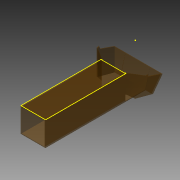
# Autodesk Inventor part: Ball Collector
Saved by Autodesk Inventor 2013 (Build 170138000, 138)
## iProperties
Created: 2014-09-14
Part Number: Ball Collector
Document SubType Name: Modeling
Designer: Family Room
Density: 1 g/cm^3
Material: Generic
Author: Family Room
Autodesk Inventor part; units mm, degrees
sketch "Sketch1" plane through (0, 0, 0) normal (0, 0, 1) x (1, 0, 0)
  line L0 (0, 0) -> (95.25, 0)
  line L1 (95.25, 0) -> (95.25, 95.25)
  line L2 (95.25, 95.25) -> (0, 95.25)
  line L3 (0, 95.25) -> (0, 0)
  line L4 (-3.175, -3.175) -> (98.425, -3.175)
  line L5 (98.425, -3.175) -> (98.425, 98.425)
  line L6 (98.425, 98.425) -> (-3.175, 98.425)
  line L7 (-3.175, 98.425) -> (-3.175, -3.175)
  dimension "d0" = 95.25
  dimension "d1" = 95.25
  dimension "d2" = 3.175
  constraints: 16 end point, 4 parallel, 2 perpendicular, 1 horizontal, 3 other
  measures "d0" distance of L2.end L1.end
  measures "d1" distance of L1.end L0.end
  measures "d2" distance between parallel lines of L7 L3
sketch "Sketch1 outline for Extrusion1" plane through (0, 0, 0) normal (0, 0, 1) x (1, 0, 0)
  line L0 (-3.175, 98.425) -> (-3.175, -3.175)
  line L1 (98.425, 98.425) -> (-3.175, 98.425)
  line L2 (-3.175, -3.175) -> (98.425, -3.175)
  line L3 (98.425, -3.175) -> (98.425, 98.425)
  line L4 (0, 95.25) -> (0, 0)
  line L5 (0, 0) -> (95.25, 0)
  line L6 (95.25, 0) -> (95.25, 95.25)
  line L7 (95.25, 95.25) -> (0, 95.25)
extrude "Extrusion1" add sketch "Sketch1 outline for Extrusion1" along normal blind 406.4
sketch "Sketch3" plane through (0, 0, 0) normal (0, 0, -1) x (-1, 0, 0)
  line L0 (0, 95.25) -> (0, 0) projected
  line L1 (0, 0) -> (-95.25, 0) projected
  line L2 (-95.25, 0) -> (-95.25, 95.25) projected
  line L3 (-95.25, 95.25) -> (0, 95.25) projected
  line L4 (3.175, -3.175) -> (-98.425, -3.175) projected
  line L5 (3.175, 98.425) -> (3.175, -3.175) projected
  line L6 (-98.425, 98.425) -> (3.175, 98.425) projected
  line L7 (-98.425, -3.175) -> (-98.425, 98.425) projected
sketch "Sketch3 outline for Extrusion2" plane through (0, 0, 0) normal (0, 0, -1) x (-1, 0, 0)
  line L0 (-98.425, 98.425) -> (-98.425, -3.175)
  line L1 (3.175, 98.425) -> (-98.425, 98.425)
  line L2 (-98.425, -3.175) -> (3.175, -3.175)
  line L3 (3.175, -3.175) -> (3.175, 98.425)
  line L4 (-95.25, 95.25) -> (0, 95.25)
  line L5 (-95.25, 0) -> (-95.25, 95.25)
  line L6 (0, 0) -> (-95.25, 0)
  line L7 (0, 95.25) -> (0, 0)
extrude "Extrusion2" cut sketch "Sketch3 outline for Extrusion2" against normal blind 50.8
sketch "Sketch4" plane through (-3.175, 98.425, 406.4) normal (0, 1, 0) x (1, 0, 0)
  line L0 (101.6, 355.6) -> (0, 355.6) projected
  line L1 (0, 355.6) -> (0, 0) projected
  line L2 (101.6, 355.6) -> (0, 355.6)
  line L3 (0, 355.6) -> (0, 266.7)
  line L4 (0, 266.7) -> (101.6, 266.7)
  line L5 (101.6, 266.7) -> (101.6, 355.6)
  point P0 (3.175, 406.4)
  dimension "d7" = 88.9
  constraints: 8 end point, 2 parallel, 1 horizontal, 1 perpendicular, 1 point on line
  measures "d7" distance of L3.end L2.end
sketch "Sketch4 outline for Extrusion3" plane through (-3.175, 98.425, 406.4) normal (0, 1, 0) x (1, 0, 0)
  line L0 (101.6, 266.7) -> (101.6, 355.6)
  line L1 (0, 266.7) -> (101.6, 266.7)
  line L2 (0, 355.6) -> (0, 266.7)
  line L3 (101.6, 355.6) -> (0, 355.6)
extrude "Extrusion3" cut sketch "Sketch4 outline for Extrusion3" against normal blind 98.425
sketch "Sketch5" plane through (0, 0, 50.8) normal (0, 0, -1) x (-1, 0, 0)
  line L0 (3.175, 0) -> (-98.425, 0)
  line L1 (-98.425, -3.175) -> (-98.425, 0)
  line L2 (3.175, 0) -> (3.175, -3.175)
  line L3 (3.175, -3.175) -> (55.29887, 140.034155)
  line L4 (3.175, -3.175) -> (155.575, -3.175) construction
  line L5 (-98.425, -3.175) -> (-150.54887, 140.034155)
  line L6 (-98.425, -3.175) -> (53.975, -3.175) construction
  line L7 (-98.425, -3.175) -> (3.175, -3.175)
  line L8 (-98.425, 98.425) -> (40.154376, 98.425)
  line L9 (-98.425, 98.425) -> (-135.404376, 98.425)
  point P0 (0, 0)
  dimension "d10" = 152.4
  dimension "d11" = 70
  dimension "d12" = 152.4
  dimension "d13" = 110
  dimension "d14" = 101.6
  constraints: 14 end point, 2 collinear, 2 equal length, 2 horizontal, 2 point on line
  measures "d10" distance of L2.end L3.end
  measures "d11" angle of L4 L3
  measures "d12" distance of L1.start L5.end
  measures "d13" angle of L6 L5
  measures "d14" distance of L1.start L8.start
sketch "Sketch5 outline for Extrusion4" plane through (0, 0, 50.8) normal (0, 0, -1) x (-1, 0, 0)
  line L0 (-98.425, 0) -> (3.175, 0)
  line L1 (-98.425, -3.175) -> (-98.425, 0)
  line L2 (-135.404376, 98.425) -> (-98.425, -3.175)
  line L3 (-98.425, 98.425) -> (-135.404376, 98.425)
  line L4 (40.154376, 98.425) -> (-98.425, 98.425)
  line L5 (3.175, -3.175) -> (40.154376, 98.425)
  line L6 (3.175, 0) -> (3.175, -3.175)
extrude "Extrusion4" add sketch "Sketch5 outline for Extrusion4" against normal blind 3.175
sketch "Sketch6" plane through (0, 0, 53.975) normal (0, 0, 1) x (1, 0, 0)
  line L0 (-3.175, -3.175) -> (-40.154376, 98.425)
  line L1 (135.404376, 98.425) -> (98.425, -3.175)
  line L2 (-40.154376, 98.425) -> (135.404376, 98.425)
  line L3 (98.425, -3.175) -> (135.404376, 98.425)
  line L4 (-40.154376, 98.425) -> (-3.175, -3.175)
  line L5 (-3.175, -3.175) -> (98.425, -3.175)
  line L6 (130.870006, 95.25) -> (96.201841, 0)
  line L7 (96.201841, 0) -> (-0.951841, 0)
  line L8 (-0.951841, 0) -> (-35.620006, 95.25)
  line L9 (130.870006, 95.25) -> (132.025611, 98.425)
  line L10 (98.964652, 7.590761) -> (101.948176, 6.504847)
  line L11 (-3.714652, 7.590761) -> (-6.698176, 6.504847)
  line L12 (-35.620006, 95.25) -> (-36.775611, 98.425)
  line L13 (135.404376, 98.425) -> (132.025611, 98.425)
  line L14 (-36.775611, 98.425) -> (-40.154376, 98.425)
  point P0 (0, 0)
  constraints: 24 end point, 5 collinear, 4 point on line, 3 perpendicular, 2 parallel, 2 other
sketch "Sketch6 outline for Extrusion5" plane through (0, 0, 53.975) normal (0, 0, 1) x (1, 0, 0)
  line L0 (101.948176, 6.504847) -> (135.404376, 98.425)
  line L1 (135.404376, 98.425) -> (132.025611, 98.425)
  line L2 (132.025611, 98.425) -> (98.964652, 7.590761)
  line L3 (98.964652, 7.590761) -> (101.948176, 6.504847)
  line L4 (-36.775611, 98.425) -> (-40.154376, 98.425)
  line L5 (-40.154376, 98.425) -> (-6.698176, 6.504847)
  line L6 (-6.698176, 6.504847) -> (-3.714652, 7.590761)
  line L7 (-3.714652, 7.590761) -> (-36.775611, 98.425)
extrude "Extrusion5" add sketch "Sketch6 outline for Extrusion5" along normal blind 82.55
sketch "Sketch7" plane through (0, 0, 406.4) normal (0, 0, 1) x (1, 0, 0)
  line L0 (0, 0) -> (0, 95.25) projected
  line L1 (0, 95.25) -> (95.25, 95.25) projected
  line L2 (95.25, 95.25) -> (95.25, 0) projected
  line L3 (95.25, 0) -> (0, 0) projected
  line L4 (-3.175, -3.175) -> (-3.175, 98.425) projected
  line L5 (98.425, -3.175) -> (-3.175, -3.175) projected
  line L6 (98.425, 98.425) -> (98.425, -3.175) projected
  line L7 (-3.175, 98.425) -> (98.425, 98.425) projected
sketch "Sketch7 outline for Extrusion6" plane through (0, 0, 406.4) normal (0, 0, 1) x (1, 0, 0)
  line L0 (98.425, 98.425) -> (-3.175, 98.425)
  line L1 (98.425, -3.175) -> (98.425, 98.425)
  line L2 (-3.175, 98.425) -> (-3.175, -3.175)
  line L3 (-3.175, -3.175) -> (98.425, -3.175)
  line L4 (95.25, 0) -> (0, 0)
  line L5 (95.25, 95.25) -> (95.25, 0)
  line L6 (0, 95.25) -> (95.25, 95.25)
  line L7 (0, 0) -> (0, 95.25)
extrude "Extrusion6" add sketch "Sketch7 outline for Extrusion6" along normal blind 88.9
ref_plane "Work Plane1" through (47.625, 0, 139.7) normal (-1, 0, 0) x (0, 0, 1)
sketch "Sketch8" plane through (98.425, 0, 139.7) normal (1, 0, 0) x (0, 0, -1)
  line L0 (85.725, -3.175) -> (-355.6, -3.175)
  line L1 (209.478818, 0) -> (209.478818, 140.094792)
  line L2 (209.478818, 140.094792) -> (0, 140.094792)
  line L3 (0, 140.094792) -> (0, 0)
  line L4 (0, 0) -> (209.478818, 0)
  point P0 (139.7, 0)
  point P1 (0, -3.175)
  constraints: 8 end point, 2 point on line, 1 parallel, 1 perpendicular
sketch "Sketch8 outline for Extrusion7" plane through (98.425, 0, 139.7) normal (1, 0, 0) x (0, 0, -1)
  line L0 (209.478818, 140.094792) -> (209.478818, 0)
  line L1 (209.478818, 0) -> (0, 0)
  line L2 (0, 0) -> (0, 140.094792)
  line L3 (0, 140.094792) -> (209.478818, 140.094792)
extrude "Extrusion7" cut sketch "Sketch8 outline for Extrusion7" along normal through all both and the other way through all
sketch "Sketch9" plane through (0, 0, 495.3) normal (0, 0, 1) x (1, 0, 0)
  line L0 (0, 95.25) -> (95.25, 95.25) projected
  line L1 (95.25, 95.25) -> (95.25, 0) projected
  line L2 (95.25, 0) -> (0, 0) projected
  line L3 (0, 0) -> (0, 95.25) projected
  line L4 (-3.175, 98.425) -> (98.425, 98.425) projected
  line L5 (-3.175, -3.175) -> (-3.175, 98.425) projected
  line L6 (98.425, -3.175) -> (-3.175, -3.175) projected
  line L7 (98.425, 98.425) -> (98.425, -3.175) projected
sketch "Sketch9 outline for Extrusion8" plane through (0, 0, 495.3) normal (0, 0, 1) x (1, 0, 0)
  line L0 (98.425, -3.175) -> (98.425, 98.425)
  line L1 (-3.175, -3.175) -> (98.425, -3.175)
  line L2 (98.425, 98.425) -> (-3.175, 98.425)
  line L3 (-3.175, 98.425) -> (-3.175, -3.175)
  line L4 (0, 0) -> (0, 95.25)
  line L5 (95.25, 0) -> (0, 0)
  line L6 (95.25, 95.25) -> (95.25, 0)
  line L7 (0, 95.25) -> (95.25, 95.25)
extrude "Extrusion8" cut sketch "Sketch9 outline for Extrusion8" against normal blind 25.4
ref_plane "Work Plane3" through (99.580605, 0, 53.975) normal (1, 0, 0) x (0, 0, -1)
sketch "Sketch11" plane through (99.580605, 0, 53.975) normal (1, 0, 0) x (0, 0, -1)
  line L0 (0, 0) -> (4.92371, 0)
  line L1 (4.92371, 0) -> (4.92371, -5.872358)
  line L2 (4.92371, -5.872358) -> (0, -5.872358)
  line L3 (0, -5.872358) -> (0, 0)
  point P0 (53.975, 0)
  constraints: 8 end point, 2 parallel, 1 horizontal, 1 perpendicular
sketch "Sketch11 outline for Extrusion9" plane through (99.580605, 0, 53.975) normal (1, 0, 0) x (0, 0, -1)
  line L0 (0, 0) -> (4.92371, 0)
  line L1 (4.92371, 0) -> (4.92371, -5.872358)
  line L2 (4.92371, -5.872358) -> (0, -5.872358)
  line L3 (0, -5.872358) -> (0, 0)
extrude "Extrusion9" cut sketch "Sketch11 outline for Extrusion9" against normal through all
sketch "Sketch12" plane through (98.425, 0, 139.7) normal (1, 0, 0) x (0, 0, -1)
  line L0 (85.725, -3.175) -> (85.725, 0)
  line L1 (85.725, 0) -> (0, 0)
  line L2 (85.725, -3.175) -> (115.308017, 107.230322)
  line L3 (85.725, -3.175) -> (200.025, -3.175) construction
  line L4 (115.308017, 107.230322) -> (112.241202, 108.052072)
  line L5 (112.241202, 108.052072) -> (81.725693, 0)
  line L6 (81.725693, 0) -> (85.725, -3.175)
  point P0 (139.7, 0)
  dimension "d29" = 114.3
  dimension "d30" = 75
  dimension "d31" = 3.175
  constraints: 10 end point, 1 equal length, 1 horizontal, 1 perpendicular, 1 point on line
  measures "d29" distance of L0.start L2.end
  measures "d30" angle of L3 L2
  measures "d31" distance of L2.end L4.end
sketch "Sketch12 outline for Extrusion10" plane through (98.425, 0, 139.7) normal (1, 0, 0) x (0, 0, -1)
  line L0 (85.725, 0) -> (85.725, -3.175)
  line L1 (81.725693, 0) -> (85.725, 0)
  line L2 (112.241202, 108.052072) -> (81.725693, 0)
  line L3 (115.308017, 107.230322) -> (112.241202, 108.052072)
  line L4 (85.725, -3.175) -> (115.308017, 107.230322)
extrude "Extrusion10" add sketch "Sketch12 outline for Extrusion10" against normal blind 101.6
sketch "Sketch13" plane through (98.425, 107.230322, 24.391983) normal (0, -0.258819, -0.9659258) x (-1, 0, 0)
  line L0 (101.6, -114.3) -> (101.6, 0)
  line L1 (0, 0) -> (101.6, 0)
  line L2 (0, -114.3) -> (0, 0)
  line L3 (101.6, -114.3) -> (0, -114.3)
  line L4 (0, -114.3) -> (101.6, -114.3)
  line L5 (101.6, -114.3) -> (130.175, -114.3)
  line L6 (130.175, -114.3) -> (160.801593, 0)
  line L7 (0, -114.3) -> (-28.575, -114.3)
  line L8 (-28.575, -114.3) -> (-59.201593, 0)
  line L9 (160.801593, 0) -> (-59.201593, 0)
  point P0 (98.425, -97.263428)
  dimension "d34" = 28.575
  dimension "d35" = 105
  dimension "d36" = 28.575
  dimension "d37" = 105
  dimension "d40" = 114.3
  constraints: 12 end point, 3 collinear, 1 parallel
  measures "d34" distance of L0.start L5.end
  measures "d35" angle of L6 L5
  measures "d36" distance of L2.start L7.end
  measures "d37" angle of L7 L8
  measures "d40" distance between parallel lines of L3 L9
sketch "Sketch13 outline for Extrusion11" plane through (98.425, 107.230322, 24.391983) normal (0, -0.258819, -0.9659258) x (-1, 0, 0)
  line L0 (-28.575, -114.3) -> (0, -114.3)
  line L1 (-59.201593, 0) -> (-28.575, -114.3)
  line L2 (0, 0) -> (-59.201593, 0)
  line L3 (0, 0) -> (0, -114.3)
  line L4 (101.6, -114.3) -> (101.6, 0)
  line L5 (160.801593, 0) -> (101.6, 0)
  line L6 (130.175, -114.3) -> (160.801593, 0)
  line L7 (101.6, -114.3) -> (130.175, -114.3)
extrude "Extrusion11" add sketch "Sketch13 outline for Extrusion11" against normal blind 3.175
sketch "Sketch14" plane through (127, -3.175, 53.975) normal (0, -0.258819, -0.9659258) x (-1, 0, 0)
  line L0 (189.376593, 114.3) -> (-30.626593, 114.3)
  line L1 (-30.626593, 114.3) -> (0, 0)
  line L2 (130.175, 0) -> (158.75, 0)
  line L3 (158.75, 0) -> (189.376593, 114.3)
  line L4 (-30.626593, 114.3) -> (0, 0)
  line L5 (0, 0) -> (158.75, 0)
  line L6 (158.75, 0) -> (189.376593, 114.3)
  line L7 (186.309778, 115.12175) -> (156.313737, 3.175)
  line L8 (156.313737, 3.175) -> (2.436263, 3.175)
  line L9 (2.436263, 3.175) -> (-27.559778, 115.12175)
  line L10 (-30.626593, 114.3) -> (-27.339591, 114.3)
  line L11 (189.376593, 114.3) -> (186.089591, 114.3)
  line L12 (0, 0) -> (28.575, 0)
  line L13 (156.313737, 3.175) -> (155.462998, 0)
  line L14 (2.436263, 3.175) -> (3.287002, 0)
  point P0 (127, 17.036572)
  dimension "d41" = 3.175
  constraints: 20 end point, 6 point on line, 5 collinear, 2 other
  measures "d41" distance between parallel lines of L2 L8
sketch "Sketch14 outline for Extrusion12" plane through (127, -3.175, 53.975) normal (0, -0.258819, -0.9659258) x (-1, 0, 0)
  line L0 (158.75, 0) -> (189.376593, 114.3)
  line L1 (189.376593, 114.3) -> (186.089591, 114.3)
  line L2 (186.089591, 114.3) -> (155.462998, 0)
  line L3 (155.462998, 0) -> (158.75, 0)
  line L4 (-27.339591, 114.3) -> (-30.626593, 114.3)
  line L5 (-30.626593, 114.3) -> (0, 0)
  line L6 (0, 0) -> (3.287002, 0)
  line L7 (3.287002, 0) -> (-27.339591, 114.3)
extrude "Extrusion12" add sketch "Sketch14 outline for Extrusion12" against normal blind 76.2
sketch "Sketch15" plane through (98.425, 98.425, 139.7) normal (0, 0, -1) x (-1, 0, 0)
  line L0 (3.175, -3.175) -> (3.175, -98.425) projected
  line L1 (0, 0) -> (3.175, 0)
  line L2 (3.175, 0) -> (3.175, -76.2)
  line L3 (3.175, -76.2) -> (0, -76.2)
  line L4 (0, -76.2) -> (0, 0)
  dimension "d44" = 76.2
  constraints: 8 end point, 2 parallel, 1 horizontal, 1 perpendicular, 1 point on line
  measures "d44" distance of L1.end L2.end
sketch "Sketch15 outline for Extrusion13" plane through (98.425, 98.425, 139.7) normal (0, 0, -1) x (-1, 0, 0)
  line L0 (3.175, 0) -> (0, 0)
  line L1 (3.175, -76.2) -> (3.175, 0)
  line L2 (0, -76.2) -> (3.175, -76.2)
  line L3 (0, 0) -> (0, -76.2)
extrude "Extrusion13" add sketch "Sketch15 outline for Extrusion13" along normal blind 2.54
loft "Loft1" add section 1 edges at (96.8375, 98.425, 137.16) (98.425, 60.325, 137.16) (96.8375, 22.225, 137.16) (95.25, 60.325, 137.16) section 2 edges at (125.356499, 16.547011, 127.578548) (142.313296, 71.749672, 112.78704) (155.983092, 126.952333, 97.995531) (139.026294, 71.749672, 112.78704)
sketch "Sketch16" plane through (95.25, 98.425, 139.7) normal (0, 0, -1) x (-1, 0, 0)
  line L0 (95.25, -98.425) -> (95.25, -3.175) projected
  line L1 (98.425, 0) -> (95.25, 0)
  line L2 (95.25, 0) -> (95.25, -76.2)
  line L3 (95.25, -76.2) -> (98.425, -76.2)
  line L4 (98.425, -76.2) -> (98.425, 0)
  dimension "d51" = 76.2
  constraints: 8 end point, 2 parallel, 1 horizontal, 1 perpendicular, 1 point on line
  measures "d51" distance of L2.end L1.end
sketch "Sketch16 outline for Extrusion14" plane through (95.25, 98.425, 139.7) normal (0, 0, -1) x (-1, 0, 0)
  line L0 (95.25, 0) -> (95.25, -76.2)
  line L1 (98.425, 0) -> (95.25, 0)
  line L2 (98.425, -76.2) -> (98.425, 0)
  line L3 (95.25, -76.2) -> (98.425, -76.2)
extrude "Extrusion14" add sketch "Sketch16 outline for Extrusion14" along normal blind 2.54
loft "Loft2" add section 1 edges at (0, 60.325, 137.16) (-1.5875, 22.225, 137.16) (-3.175, 60.325, 137.16) (-1.5875, 98.425, 137.16) section 2 edges at (-43.776294, 71.749672, 112.78704) (-60.733092, 126.952333, 97.995531) (-47.063296, 71.749672, 112.78704) (-30.106499, 16.547011, 127.578548)
ref_plane "Work Plane4" through (-62.376593, 126.952333, 97.995531) normal (-1, 0, 0) x (0, 0, 1)
sketch "Sketch17" plane through (-62.376593, 126.952333, 97.995531) normal (-1, 0, 0) x (0, 0, 1)
  line L0 (0, 0) -> (39.581959, 0)
  line L1 (39.581959, 0) -> (39.581959, -28.813692)
  line L2 (39.581959, -28.813692) -> (0, -28.813692)
  line L3 (0, -28.813692) -> (-21.532096, -5.667761)
  line L4 (-21.532096, -5.667761) -> (0, 0)
  point P0 (-97.995531, -126.952333)
  constraints: 10 end point, 1 horizontal, 1 parallel, 1 perpendicular
sketch "Sketch17 outline for Extrusion15" plane through (-62.376593, 126.952333, 97.995531) normal (-1, 0, 0) x (0, 0, 1)
  line L0 (0, 0) -> (39.581959, 0)
  line L1 (39.581959, 0) -> (39.581959, -28.813692)
  line L2 (39.581959, -28.813692) -> (0, -28.813692)
  line L3 (0, -28.813692) -> (-21.532096, -5.667761)
  line L4 (-21.532096, -5.667761) -> (0, 0)
extrude "Extrusion15" cut sketch "Sketch17 outline for Extrusion15" against normal through all
ref_plane "Work Plane5" through (-62.376593, 121.203127, 76.539202) normal (-1, 0, 0) x (0, 0, 1)
sketch "Sketch18" plane through (-62.376593, 121.203127, 76.539202) normal (-1, 0, 0) x (0, 0, 1)
  line L0 (19.452148, -31.292775) -> (-58.109978, -57.697076)
  line L1 (19.452148, -31.292775) -> (24.815614, 22.153396)
  line L2 (24.815614, 22.153396) -> (-54.454563, 58.685988)
  line L3 (-58.109978, -57.697076) -> (-54.454563, 58.685988)
  point P0 (-76.539202, -121.203127)
  constraints: 8 end point
sketch "Sketch18 outline for Extrusion16" plane through (-62.376593, 121.203127, 76.539202) normal (-1, 0, 0) x (0, 0, 1)
  line L0 (19.452148, -31.292775) -> (-58.109978, -57.697076)
  line L1 (-58.109978, -57.697076) -> (-54.454563, 58.685988)
  line L2 (-54.454563, 58.685988) -> (24.815614, 22.153396)
  line L3 (24.815614, 22.153396) -> (19.452148, -31.292775)
extrude "Extrusion16" cut sketch "Sketch18 outline for Extrusion16" against normal through all
sketch "Sketch19" plane through (0, 98.425, 139.7) normal (0, 1, 0) x (1, 0, 0)
  line L0 (-3.175, 2.12251) -> (-3.175, -330.2)
  line L1 (-3.175, -330.2) -> (98.425, -330.2)
  line L2 (98.425, 2.12251) -> (98.425, -330.2)
  line L3 (95.25, 0) -> (0, 0)
  line L4 (-3.175, 0) -> (12.827, 0)
  line L5 (12.827, 0) -> (12.827, -38.1)
  line L6 (98.425, 0) -> (82.423, 0)
  line L7 (82.423, 0) -> (82.423, -38.1)
  line L8 (-3.175, -330.2) -> (12.827, -330.2)
  line L9 (98.425, -330.2) -> (82.423, -330.2)
  line L10 (82.423, -330.2) -> (82.423, -254)
  line L11 (12.827, -330.2) -> (12.827, -254)
  point P0 (0, 139.7)
  dimension "d62" = 16.002
  dimension "d63" = 38.1
  dimension "d64" = 16.002
  dimension "d65" = 76.2
  dimension "d66" = 76.2
  constraints: 16 end point, 7 point on line, 4 coincident, 3 perpendicular, 1 parallel
  measures "d62" distance of L4.start L4.end
  measures "d63" distance of L4.end L5.end
  measures "d64" distance of L6.start L6.end
  measures "d65" distance of L9.end L10.end
  measures "d66" distance of L8.end L11.end
hole "Hole1" at (12.827, 98.425, 177.8) at (82.423, 98.425, 177.8) at (12.827, 98.425, 393.7) at (82.423, 98.425, 393.7) direction (0, -1, 0) diameter 7.62 depth 25.4 tip angle 118
equation "\"d0\" = d1"
body "Solid1"
